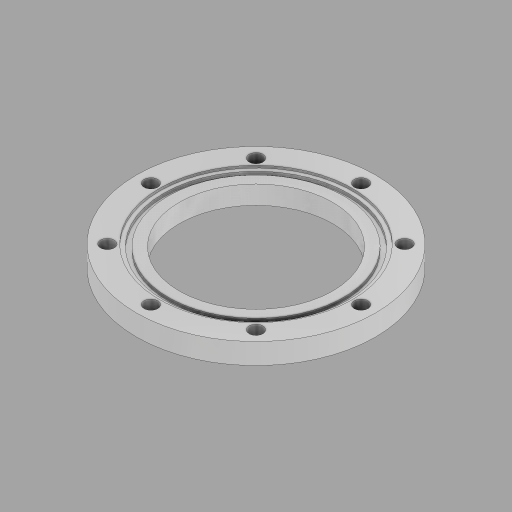
# Autodesk Inventor part: CollarRingTop
Saved by Autodesk Inventor 2024 (Build 280153020, 153B)
## iProperties
Created: 2023-10-25
Part Number: CollarRingTop
Material: Stainless Steel
Document SubType Name: Modeling
Designer: schanen
Density: 8 g/cm^3
Appearance: Polished - Small Pyramid Knurl
Author: schanen
Autodesk Inventor part; units mm, degrees
ref_plane "YZ Plane" through (0, 0, 0) normal (1, 0, 0) x (0, 1, 0)
ref_plane "XZ Plane" through (0, 0, 0) normal (0, 1, 0) x (-1, 0, 0)
ref_plane "XY Plane" through (0, 0, 0) normal (0, 0, 1) x (1, 0, 0)
sketch "Sketch1" plane through (0, 0, 0) normal (0, 0, 1) x (1, 0, 0)
  line L0 (-103.5, 0) -> (-103.5, 18)
  line L1 (-103.5, 18) -> (-83.5, 18)
  line L2 (-83.5, 18) -> (-83.5, 16)
  line L3 (-83.5, 16) -> (-80, 16)
  line L4 (-80, 16) -> (-80, 13.25)
  line L5 (-80, 13.25) -> (-76, 13.25)
  line L6 (-76, 13.25) -> (-76, 16)
  line L7 (-76, 16) -> (-66.5, 16)
  line L8 (-66.5, 16) -> (-66.5, 0)
  line L9 (-66.5, 0) -> (-103.5, 0)
  line L10 (0, -3.6) -> (0, 21.6) projected
  point P0 (0, 0)
  dimension "d0" = 103.5
  dimension "d1" = 20
  dimension "d2" = 4
  dimension "d3" = 76
  dimension "d4" = 66.5
  dimension "d5" = 18
  dimension "d6" = 2
  dimension "d7" = 2.75
  constraints: 20 end point, 8 perpendicular, 2 point on line, 1 horizontal alignment, 1 vertical
  measures "d0" distance from line of point (0, 0) L0
  measures "d1" distance between parallel lines of L0 L2
  measures "d2" distance of L4.end L5.end
  measures "d3" distance from line of point (0, 0) L6
  measures "d4" distance from line of point (0, 0) L8
  measures "d5" distance of L0.start L0.end
  measures "d6" distance of L1.end L2.end
  measures "d7" distance of L3.end L4.end
revolve "Revolution1" add sketch "Sketch1" angle 360 about axis through (0, -10, 0) along (0, 1, 0)
sketch "Sketch2" plane through (0, 18, 0) normal (0, 1, 0) x (1, 0, 0)
  circle A0 centre (0, 0) radius 103.5 projected
  point P0 (0, 91)
  dimension "d9" = 91
  constraints: 1 vertical alignment
  measures "d9" distance of point (0, 0) point (0, 91)
hole "Hole1" at (0, 18, -91) direction (0, -1, 0) diameter 12 end through all
pattern_circular "Circular Pattern1" count 8 over 360 about axis through (0, 8, 0) along (0, 1, 0) of "Hole1"
body "Solid1"
